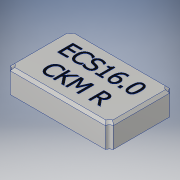
# Autodesk Inventor part: Crystal_ECX-42
Saved by Autodesk Inventor 2018 (Build 220112000, 112)
## iProperties
Created: 2016-08-15
Part Number: Crystal_ECX-42
Material: Aluminum 6061
Document SubType Name: Modeling
Designer: Bradley
Density: 2.7 g/cm^3
Appearance: Aluminum - Flat
Author: Bradley
Autodesk Inventor part; units mm, degrees
ref_plane "YZ Plane" through (0, 0, 0) normal (1, 0, 0) x (0, 1, 0)
ref_plane "XZ Plane" through (0, 0, 0) normal (0, 1, 0) x (-1, 0, 0)
ref_plane "XY Plane" through (0, 0, 0) normal (0, 0, 1) x (1, 0, 0)
sketch "Sketch1" plane through (0, 0, 0) normal (0, 1, 0) x (-1, 0, 0)
  line L0 (-2, 1.25) -> (2, 1.25)
  line L1 (2, 1.25) -> (2, -1.25)
  line L2 (2, -1.25) -> (-2, -1.25)
  line L3 (-2, -1.25) -> (-2, 1.25)
  line L4 (-2, 1.25) -> (2, -1.25) construction
  line L5 (2, 1.25) -> (-2, -1.25) construction
  arc A0 (2, -1.1) -> (1.85, -1.25) centre (2, -1.25) ccw
  arc A1 (-1.85, -1.25) -> (-2, -1.1) centre (-2, -1.25) ccw
  arc A2 (-2, 1.1) -> (-1.85, 1.25) centre (-2, 1.25) ccw
  arc A3 (1.85, 1.25) -> (2, 1.1) centre (2, 1.25) ccw
  point P0 (0, 0)
  dimension "d0" = 4
  dimension "d1" = 2.5
  dimension "d4" = 0.15
  constraints: 12 end point, 8 point on circle, 8 point on line, 4 centre point, 4 coincident, 3 equal radius, 2 midpoint, 2 parallel, 1 horizontal, 1 perpendicular
  measures "d0" distance of L1.end L2.end
  measures "d1" distance of L0.end L1.end
  measures "d4" radius of A0
extrude "Extrusion1" add sketch "Sketch1" along normal mid plane 0.9 contours L0 A3 L1 A0 L2 A1 L3 A2
chamfer "Chamfer1" distance 0.1 angle 45 8 edges at (0, 0.45, 1.25) (-1.8939, 0.45, 1.1439) (-2, 0.45, 0) (-1.8939, 0.45, -1.1439) (0, 0.45, -1.25) (1.8939, 0.45, -1.1439) (2, 0.45, 0) (1.8939, 0.45, 1.1439)
sketch "Sketch2" plane through (0, -0.45, 0) normal (0, -1, 0) x (1, 0, 0)
  line L0 (-2, 1.1) -> (-2, -1.1) projected
  arc A0 (-1.85, -1.25) -> (-2, -1.1) centre (-2, -1.25) ccw projected
  line L1 (-1.85, -1.25) -> (1.85, -1.25) projected
  arc A1 (2, -1.1) -> (1.85, -1.25) centre (2, -1.25) ccw projected
  line L2 (2, -1.1) -> (2, 1.1) projected
  arc A2 (1.85, 1.25) -> (2, 1.1) centre (2, 1.25) ccw projected
  line L3 (1.85, 1.25) -> (-1.85, 1.25) projected
  arc A3 (-2, 1.1) -> (-1.85, 1.25) centre (-2, 1.25) ccw projected
  arc A4 (-1.85, -1.25) -> (-2, -1.1) centre (-2, -1.25) ccw projected
  line L4 (-1.9612, -1.1051) -> (-1.9, -1.0439)
  line L5 (-1.9, 1.0439) -> (-1.9612, 1.1051)
  arc A5 (-2, 1.1) -> (-1.85, 1.25) centre (-2, 1.25) ccw projected
  line L6 (-1.8551, 1.2112) -> (-1.7939, 1.15)
  line L7 (-1.7939, 1.15) -> (-1, 1.15)
  line L8 (-1, -1.15) -> (-1.7939, -1.15)
  line L9 (-1.7939, -1.15) -> (-1.8551, -1.2112)
  arc A6 (1.85, 1.25) -> (2, 1.1) centre (2, 1.25) ccw projected
  line L10 (1.8551, 1.2112) -> (1.7939, 1.15)
  line L11 (1.7939, 1.15) -> (1, 1.15)
  line L12 (1, -1.15) -> (1.7939, -1.15)
  line L13 (1.7939, -1.15) -> (1.8551, -1.2112)
  arc A7 (2, -1.1) -> (1.85, -1.25) centre (2, -1.25) ccw projected
  line L14 (1.9612, -1.1051) -> (1.9, -1.0439)
  line L15 (1.9, 1.0439) -> (1.9612, 1.1051)
  line L16 (-2, 1.25) -> (-1.8939, 1.1439) construction
  line L17 (1.85, 1.25) -> (-1.85, 1.25) construction
  line L18 (-2, -1.25) -> (-1.8939, -1.1439) construction
  line L19 (-1.9, 1.0439) -> (-1.9, 0.35)
  line L20 (-1.9, 0.35) -> (-1, 0.35)
  line L21 (-1, 0.35) -> (-1, 1.15)
  line L22 (-1.9, -1.0439) -> (-1.9, -0.35)
  line L23 (-1.9, -0.35) -> (-1, -0.35)
  line L24 (-1, -0.35) -> (-1, -1.15)
  line L25 (1.9, -1.0439) -> (1.9, -0.35)
  line L26 (1.9, -0.35) -> (1, -0.35)
  line L27 (1, -0.35) -> (1, -1.15)
  line L28 (1.9, 1.0439) -> (1.9, 0.35)
  line L29 (1.9, 0.35) -> (1, 0.35)
  line L30 (1, 1.15) -> (1, 0.35)
  point P0 (0, 0)
  dimension "d9" = 0.15
  dimension "d15" = 2
  dimension "d16" = 0.7
  dimension "d17" = 0.8
  constraints: 52 end point, 15 equal length, 15 point on circle, 9 point on line, 8 parallel, 8 perpendicular, 1 collinear, 1 vertical, 1 other
  measures "d9" distance between parallel lines of L5 L6
  measures "d15" distance between parallel lines of L30 L21
  measures "d16" distance between parallel lines of L26 L29
  measures "d17" distance of L11.end L29.end
sketch "Sketch3" plane through (0, 0.45, 0) normal (0, 1, 0) x (1, 0, 0)
  line L0 (-1.7709, 1.15) -> (1.7709, 1.15) projected
  arc A0 (-1.9, 1.0209) -> (-1.7709, 1.15) centre (-2, 1.25) ccw projected
  line L1 (-1.9, -1.0209) -> (-1.9, 1.0209) projected
  arc A1 (-1.7709, -1.15) -> (-1.9, -1.0209) centre (-2, -1.25) ccw projected
  line L2 (1.7709, -1.15) -> (-1.7709, -1.15) projected
  arc A2 (1.9, -1.0209) -> (1.7709, -1.15) centre (2, -1.25) ccw projected
  line L3 (1.9, 1.0209) -> (1.9, -1.0209) projected
  arc A3 (1.7709, 1.15) -> (1.9, 1.0209) centre (2, 1.25) ccw projected
  line L4 (1.9, 1.0209) -> (1.9, -1.0209) construction
  line L5 (1.9, 0.1868) -> (-1.9, 0.1868) construction
  line L6 (-1.4485, 0.1868) -> (-1.4485, 0.7868)
  line L7 (-1.4485, 0.7868) -> (-1.0731, 0.7868)
  line L8 (-1.0731, 0.7868) -> (-1.0731, 0.7158)
  line L9 (-1.0731, 0.7158) -> (-1.3687, 0.7158)
  line L10 (-1.3687, 0.7158) -> (-1.3687, 0.5514)
  line L11 (-1.3687, 0.5514) -> (-1.093, 0.5514)
  line L12 (-1.093, 0.5514) -> (-1.093, 0.4804)
  line L13 (-1.093, 0.4804) -> (-1.3687, 0.4804)
  line L14 (-1.3687, 0.4804) -> (-1.3687, 0.2577)
  line L15 (-1.3687, 0.2577) -> (-1.0731, 0.2577)
  line L16 (-1.0731, 0.2577) -> (-1.0731, 0.1868)
  line L17 (-1.0731, 0.1868) -> (-1.4485, 0.1868)
  spline S0 degree 2 poles (-0.7512, 0.1761) (-0.8096, 0.1761) (-0.9083, 0.2154) (-0.9442, 0.2548) knots 0 0 0 1 2 2 2
  spline S1 degree 2 poles (-0.9442, 0.2548) (-0.9802, 0.2937) (-1.0196, 0.4104) (-1.0196, 0.4863) knots 0 0 0 1 2 2 2
  spline S2 degree 2 poles (-1.0196, 0.4863) (-1.0196, 0.5616) (-0.9812, 0.6735) (-0.9447, 0.7148) knots 0 0 0 1 2 2 2
  spline S3 degree 2 poles (-0.9447, 0.7148) (-0.9088, 0.7552) (-0.8105, 0.7975) (-0.7498, 0.7975) knots 0 0 0 1 2 2 2
  spline S4 degree 2 poles (-0.7498, 0.7975) (-0.7196, 0.7975) (-0.6666, 0.7887) (-0.6442, 0.7819) knots 0 0 0 1 2 2 2
  spline S5 degree 2 poles (-0.6442, 0.7819) (-0.6248, 0.7756) (-0.5844, 0.7576) (-0.5645, 0.7469) knots 0 0 0 1 2 2 2
  line L18 (-0.5645, 0.7469) -> (-0.5645, 0.6506)
  line L19 (-0.5645, 0.6506) -> (-0.5708, 0.6506)
  spline S6 degree 2 poles (-0.5708, 0.6506) (-0.5815, 0.6603) (-0.6146, 0.6876) (-0.6384, 0.7007) knots 0 0 0 1 2 2 2
  spline S7 degree 2 poles (-0.6384, 0.7007) (-0.6613, 0.7133) (-0.7152, 0.7294) (-0.7502, 0.7294) knots 0 0 0 1 2 2 2
  spline S8 degree 2 poles (-0.7502, 0.7294) (-0.7887, 0.7294) (-0.8572, 0.6978) (-0.883, 0.6676) knots 0 0 0 1 2 2 2
  spline S9 degree 2 poles (-0.883, 0.6676) (-0.9083, 0.637) (-0.9365, 0.5441) (-0.9365, 0.4863) knots 0 0 0 1 2 2 2
  spline S10 degree 2 poles (-0.9365, 0.4863) (-0.9365, 0.4245) (-0.9068, 0.3355) (-0.881, 0.3049) knots 0 0 0 1 2 2 2
  spline S11 degree 2 poles (-0.881, 0.3049) (-0.8558, 0.2752) (-0.7882, 0.2451) (-0.7502, 0.2451) knots 0 0 0 1 2 2 2
  spline S12 degree 2 poles (-0.7502, 0.2451) (-0.7157, 0.2451) (-0.6569, 0.2621) (-0.634, 0.2748) knots 0 0 0 1 2 2 2
  spline S13 degree 2 poles (-0.634, 0.2748) (-0.6122, 0.2874) (-0.5796, 0.3137) (-0.5703, 0.3229) knots 0 0 0 1 2 2 2
  line L20 (-0.5703, 0.3229) -> (-0.5645, 0.3229)
  line L21 (-0.5645, 0.3229) -> (-0.5645, 0.2276)
  spline S14 degree 2 poles (-0.5645, 0.2276) (-0.5844, 0.2184) (-0.6194, 0.2013) (-0.6442, 0.1936) knots 0 0 0 1 2 2 2
  spline S15 degree 2 poles (-0.6442, 0.1936) (-0.6705, 0.1848) (-0.7152, 0.1761) (-0.7512, 0.1761) knots 0 0 0 1 2 2 2
  spline S16 degree 2 poles (-0.3229, 0.1761) (-0.388, 0.1761) (-0.4794, 0.2033) (-0.5198, 0.2227) knots 0 0 0 1 2 2 2
  line L22 (-0.5198, 0.2227) -> (-0.5198, 0.3229)
  line L23 (-0.5198, 0.3229) -> (-0.5139, 0.3229)
  spline S17 degree 2 poles (-0.5139, 0.3229) (-0.4746, 0.2859) (-0.3749, 0.2451) (-0.3287, 0.2451) knots 0 0 0 1 2 2 2
  spline S18 degree 2 poles (-0.3287, 0.2451) (-0.2626, 0.2451) (-0.195, 0.3) (-0.195, 0.3453) knots 0 0 0 1 2 2 2
  spline S19 degree 2 poles (-0.195, 0.3453) (-0.195, 0.3812) (-0.2305, 0.426) (-0.2689, 0.4372) knots 0 0 0 1 2 2 2
  spline S20 degree 2 poles (-0.2689, 0.4372) (-0.2966, 0.4449) (-0.3428, 0.4556) (-0.3773, 0.4644) knots 0 0 0 1 2 2 2
  spline S21 degree 2 poles (-0.3773, 0.4644) (-0.4084, 0.4727) (-0.4575, 0.4975) (-0.4765, 0.5174) knots 0 0 0 1 2 2 2
  spline S22 degree 2 poles (-0.4765, 0.5174) (-0.495, 0.5373) (-0.5154, 0.5908) (-0.5154, 0.6258) knots 0 0 0 1 2 2 2
  spline S23 degree 2 poles (-0.5154, 0.6258) (-0.5154, 0.6988) (-0.4016, 0.7975) (-0.3136, 0.7975) knots 0 0 0 1 2 2 2
  spline S24 degree 2 poles (-0.3136, 0.7975) (-0.263, 0.7975) (-0.1736, 0.7775) (-0.1352, 0.7586) knots 0 0 0 1 2 2 2
  line L24 (-0.1352, 0.7586) -> (-0.1352, 0.6633)
  line L25 (-0.1352, 0.6633) -> (-0.141, 0.6633)
  spline S25 degree 2 poles (-0.141, 0.6633) (-0.1697, 0.6895) (-0.2592, 0.7284) (-0.3083, 0.7284) knots 0 0 0 1 2 2 2
  spline S26 degree 2 poles (-0.3083, 0.7284) (-0.3637, 0.7284) (-0.4323, 0.6764) (-0.4323, 0.6341) knots 0 0 0 1 2 2 2
  spline S27 degree 2 poles (-0.4323, 0.6341) (-0.4323, 0.5962) (-0.3919, 0.5509) (-0.354, 0.5407) knots 0 0 0 1 2 2 2
  spline S28 degree 2 poles (-0.354, 0.5407) (-0.3287, 0.5339) (-0.2553, 0.5164) (-0.231, 0.5091) knots 0 0 0 1 2 2 2
  spline S29 degree 2 poles (-0.231, 0.5091) (-0.1692, 0.4902) (-0.1118, 0.4138) (-0.1118, 0.3579) knots 0 0 0 1 2 2 2
  spline S30 degree 2 poles (-0.1118, 0.3579) (-0.1118, 0.3224) (-0.1405, 0.2543) (-0.1663, 0.2305) knots 0 0 0 1 2 2 2
  spline S31 degree 2 poles (-0.1663, 0.2305) (-0.195, 0.2043) (-0.2679, 0.1761) (-0.3229, 0.1761) knots 0 0 0 1 2 2 2
  line L26 (0.2922, 0.1868) -> (-0.0005, 0.1868)
  line L27 (-0.0005, 0.1868) -> (-0.0005, 0.248)
  line L28 (-0.0005, 0.248) -> (0.1084, 0.248)
  line L29 (0.1084, 0.248) -> (0.1084, 0.6501)
  line L30 (0.1084, 0.6501) -> (-0.0005, 0.6501)
  line L31 (-0.0005, 0.6501) -> (-0.0005, 0.7051)
  spline S32 degree 2 poles (-0.0005, 0.7051) (0.0613, 0.7051) (0.1196, 0.7401) (0.1235, 0.7887) knots 0 0 0 1 2 2 2
  line L32 (0.1235, 0.7887) -> (0.1857, 0.7887)
  line L33 (0.1857, 0.7887) -> (0.1857, 0.248)
  line L34 (0.1857, 0.248) -> (0.2922, 0.248)
  line L35 (0.2922, 0.248) -> (0.2922, 0.1868)
  spline S33 degree 2 poles (0.7818, 0.3812) (0.7818, 0.3351) (0.7512, 0.2568) (0.7254, 0.2305) knots 0 0 0 1 2 2 2
  spline S34 degree 2 poles (0.7254, 0.2305) (0.6987, 0.2028) (0.6316, 0.1741) (0.5912, 0.1741) knots 0 0 0 1 2 2 2
  spline S35 degree 2 poles (0.5912, 0.1741) (0.5509, 0.1741) (0.4843, 0.2013) (0.459, 0.2286) knots 0 0 0 1 2 2 2
  spline S36 degree 2 poles (0.459, 0.2286) (0.4279, 0.2611) (0.3929, 0.3705) (0.3929, 0.4503) knots 0 0 0 1 2 2 2
  spline S37 degree 2 poles (0.3929, 0.4503) (0.3929, 0.5286) (0.425, 0.6545) (0.4585, 0.7012) knots 0 0 0 1 2 2 2
  spline S38 degree 2 poles (0.4585, 0.7012) (0.4911, 0.7469) (0.5942, 0.7979) (0.6618, 0.7979) knots 0 0 0 1 2 2 2
  spline S39 degree 2 poles (0.6618, 0.7979) (0.6817, 0.7979) (0.7167, 0.794) (0.7298, 0.7897) knots 0 0 0 1 2 2 2
  line L36 (0.7298, 0.7897) -> (0.7298, 0.7124)
  line L37 (0.7298, 0.7124) -> (0.7264, 0.7124)
  spline S40 degree 2 poles (0.7264, 0.7124) (0.7152, 0.7182) (0.6744, 0.7284) (0.6511, 0.7284) knots 0 0 0 1 2 2 2
  spline S41 degree 2 poles (0.6511, 0.7284) (0.5762, 0.7284) (0.4843, 0.6273) (0.4755, 0.5281) knots 0 0 0 1 2 2 2
  spline S42 degree 2 poles (0.4755, 0.5281) (0.5042, 0.548) (0.5645, 0.5699) (0.6005, 0.5699) knots 0 0 0 1 2 2 2
  spline S43 degree 2 poles (0.6005, 0.5699) (0.6355, 0.5699) (0.688, 0.5558) (0.7167, 0.5344) knots 0 0 0 1 2 2 2
  spline S44 degree 2 poles (0.7167, 0.5344) (0.7498, 0.5096) (0.7818, 0.4328) (0.7818, 0.3812) knots 0 0 0 1 2 2 2
  spline S45 degree 2 poles (0.7002, 0.3778) (0.7002, 0.4148) (0.6807, 0.4649) (0.6593, 0.4824) knots 0 0 0 1 2 2 2
  spline S46 degree 2 poles (0.6593, 0.4824) (0.6433, 0.495) (0.6034, 0.5033) (0.5825, 0.5033) knots 0 0 0 1 2 2 2
  spline S47 degree 2 poles (0.5825, 0.5033) (0.5543, 0.5033) (0.5013, 0.4863) (0.4755, 0.4702) knots 0 0 0 1 2 2 2
  spline S48 degree 2 poles (0.4755, 0.4702) (0.475, 0.4615) (0.4741, 0.4449) (0.4741, 0.4323) knots 0 0 0 1 2 2 2
  spline S49 degree 2 poles (0.4741, 0.4323) (0.4741, 0.3701) (0.4984, 0.2937) (0.5169, 0.2738) knots 0 0 0 1 2 2 2
  spline S50 degree 2 poles (0.5169, 0.2738) (0.5339, 0.2548) (0.5708, 0.2398) (0.5917, 0.2398) knots 0 0 0 1 2 2 2
  spline S51 degree 2 poles (0.5917, 0.2398) (0.6404, 0.2398) (0.7002, 0.3088) (0.7002, 0.3778) knots 0 0 0 1 2 2 2
  line L38 (0.9817, 0.1868) -> (0.8854, 0.1868)
  line L39 (0.8854, 0.1868) -> (0.8854, 0.3015)
  line L40 (0.8854, 0.3015) -> (0.9817, 0.3015)
  line L41 (0.9817, 0.3015) -> (0.9817, 0.1868)
  spline S52 degree 2 poles (1.4762, 0.4868) (1.4762, 0.3253) (1.3823, 0.1741) (1.2846, 0.1741) knots 0 0 0 1 2 2 2
  spline S53 degree 2 poles (1.2846, 0.1741) (1.1854, 0.1741) (1.0925, 0.3282) (1.0925, 0.4863) knots 0 0 0 1 2 2 2
  spline S54 degree 2 poles (1.0925, 0.4863) (1.0925, 0.6487) (1.1864, 0.7989) (1.2846, 0.7989) knots 0 0 0 1 2 2 2
  spline S55 degree 2 poles (1.2846, 0.7989) (1.3833, 0.7989) (1.4762, 0.6433) (1.4762, 0.4868) knots 0 0 0 1 2 2 2
  spline S56 degree 2 poles (1.3731, 0.3039) (1.3848, 0.3336) (1.3945, 0.425) (1.3945, 0.4868) knots 0 0 0 1 2 2 2
  spline S57 degree 2 poles (1.3945, 0.4868) (1.3945, 0.5485) (1.3848, 0.6394) (1.3726, 0.6701) knots 0 0 0 1 2 2 2
  spline S58 degree 2 poles (1.3726, 0.6701) (1.3605, 0.7007) (1.3182, 0.7323) (1.2846, 0.7323) knots 0 0 0 1 2 2 2
  spline S59 degree 2 poles (1.2846, 0.7323) (1.2511, 0.7323) (1.2078, 0.7007) (1.1951, 0.6691) knots 0 0 0 1 2 2 2
  spline S60 degree 2 poles (1.1951, 0.6691) (1.183, 0.6385) (1.1742, 0.5451) (1.1742, 0.4863) knots 0 0 0 1 2 2 2
  spline S61 degree 2 poles (1.1742, 0.4863) (1.1742, 0.4231) (1.182, 0.3385) (1.1947, 0.3054) knots 0 0 0 1 2 2 2
  spline S62 degree 2 poles (1.1947, 0.3054) (1.2063, 0.2743) (1.2496, 0.2407) (1.2846, 0.2407) knots 0 0 0 1 2 2 2
  spline S63 degree 2 poles (1.2846, 0.2407) (1.3177, 0.2407) (1.3609, 0.2723) (1.3731, 0.3039) knots 0 0 0 1 2 2 2
  spline S64 degree 2 poles (-0.8981, -0.8128) (-0.9564, -0.8128) (-1.0551, -0.7734) (-1.0911, -0.734) knots 0 0 0 1 2 2 2
  spline S65 degree 2 poles (-1.0911, -0.734) (-1.1271, -0.6951) (-1.1665, -0.5785) (-1.1665, -0.5026) knots 0 0 0 1 2 2 2
  spline S66 degree 2 poles (-1.1665, -0.5026) (-1.1665, -0.4272) (-1.128, -0.3154) (-1.0916, -0.2741) knots 0 0 0 1 2 2 2
  spline S67 degree 2 poles (-1.0916, -0.2741) (-1.0556, -0.2337) (-0.9574, -0.1914) (-0.8966, -0.1914) knots 0 0 0 1 2 2 2
  spline S68 degree 2 poles (-0.8966, -0.1914) (-0.8665, -0.1914) (-0.8135, -0.2002) (-0.7911, -0.207) knots 0 0 0 1 2 2 2
  spline S69 degree 2 poles (-0.7911, -0.207) (-0.7716, -0.2133) (-0.7313, -0.2313) (-0.7113, -0.242) knots 0 0 0 1 2 2 2
  line L42 (-0.7113, -0.242) -> (-0.7113, -0.3383)
  line L43 (-0.7113, -0.3383) -> (-0.7177, -0.3383)
  spline S70 degree 2 poles (-0.7177, -0.3383) (-0.7284, -0.3285) (-0.7614, -0.3013) (-0.7853, -0.2882) knots 0 0 0 1 2 2 2
  spline S71 degree 2 poles (-0.7853, -0.2882) (-0.8081, -0.2755) (-0.8621, -0.2595) (-0.8971, -0.2595) knots 0 0 0 1 2 2 2
  spline S72 degree 2 poles (-0.8971, -0.2595) (-0.9355, -0.2595) (-1.0041, -0.2911) (-1.0298, -0.3212) knots 0 0 0 1 2 2 2
  spline S73 degree 2 poles (-1.0298, -0.3212) (-1.0551, -0.3519) (-1.0833, -0.4447) (-1.0833, -0.5026) knots 0 0 0 1 2 2 2
  spline S74 degree 2 poles (-1.0833, -0.5026) (-1.0833, -0.5644) (-1.0536, -0.6533) (-1.0279, -0.684) knots 0 0 0 1 2 2 2
  spline S75 degree 2 poles (-1.0279, -0.684) (-1.0026, -0.7136) (-0.935, -0.7438) (-0.8971, -0.7438) knots 0 0 0 1 2 2 2
  spline S76 degree 2 poles (-0.8971, -0.7438) (-0.8626, -0.7438) (-0.8037, -0.7267) (-0.7809, -0.7141) knots 0 0 0 1 2 2 2
  spline S77 degree 2 poles (-0.7809, -0.7141) (-0.759, -0.7015) (-0.7264, -0.6752) (-0.7172, -0.666) knots 0 0 0 1 2 2 2
  line L44 (-0.7172, -0.666) -> (-0.7113, -0.666)
  line L45 (-0.7113, -0.666) -> (-0.7113, -0.7613)
  spline S78 degree 2 poles (-0.7113, -0.7613) (-0.7313, -0.7705) (-0.7663, -0.7875) (-0.7911, -0.7953) knots 0 0 0 1 2 2 2
  spline S79 degree 2 poles (-0.7911, -0.7953) (-0.8173, -0.8041) (-0.8621, -0.8128) (-0.8981, -0.8128) knots 0 0 0 1 2 2 2
  line L46 (-0.1994, -0.8021) -> (-0.3029, -0.8021)
  line L47 (-0.3029, -0.8021) -> (-0.5222, -0.523)
  line L48 (-0.5222, -0.523) -> (-0.5572, -0.5624)
  line L49 (-0.5572, -0.5624) -> (-0.5572, -0.8021)
  line L50 (-0.5572, -0.8021) -> (-0.637, -0.8021)
  line L51 (-0.637, -0.8021) -> (-0.637, -0.2021)
  line L52 (-0.637, -0.2021) -> (-0.5572, -0.2021)
  line L53 (-0.5572, -0.2021) -> (-0.5572, -0.4778)
  line L54 (-0.5572, -0.4778) -> (-0.3112, -0.2021)
  line L55 (-0.3112, -0.2021) -> (-0.2139, -0.2021)
  line L56 (-0.2139, -0.2021) -> (-0.4624, -0.47)
  line L57 (-0.4624, -0.47) -> (-0.1994, -0.8021)
  line L58 (0.3627, -0.8021) -> (0.283, -0.8021)
  line L59 (0.283, -0.8021) -> (0.283, -0.2853)
  line L60 (0.283, -0.2853) -> (0.1264, -0.6368)
  line L61 (0.1264, -0.6368) -> (0.0778, -0.6368)
  line L62 (0.0778, -0.6368) -> (-0.0773, -0.2853)
  line L63 (-0.0773, -0.2853) -> (-0.0773, -0.8021)
  line L64 (-0.0773, -0.8021) -> (-0.1517, -0.8021)
  line L65 (-0.1517, -0.8021) -> (-0.1517, -0.2021)
  line L66 (-0.1517, -0.2021) -> (-0.0428, -0.2021)
  line L67 (-0.0428, -0.2021) -> (0.107, -0.5361)
  line L68 (0.107, -0.5361) -> (0.2519, -0.2021)
  line L69 (0.2519, -0.2021) -> (0.3627, -0.2021)
  line L70 (0.3627, -0.2021) -> (0.3627, -0.8021)
  line L71 (1.2063, -0.8021) -> (1.1028, -0.8021)
  line L72 (1.1028, -0.8021) -> (0.9131, -0.5634)
  line L73 (0.9131, -0.5634) -> (0.8217, -0.5634)
  line L74 (0.8217, -0.5634) -> (0.8217, -0.8021)
  line L75 (0.8217, -0.8021) -> (0.742, -0.8021)
  line L76 (0.742, -0.8021) -> (0.742, -0.2021)
  line L77 (0.742, -0.2021) -> (0.8966, -0.2021)
  spline S80 degree 2 poles (0.8966, -0.2021) (0.9481, -0.2021) (1.0177, -0.2133) (1.0493, -0.2337) knots 0 0 0 1 2 2 2
  spline S81 degree 2 poles (1.0493, -0.2337) (1.0809, -0.2541) (1.1173, -0.3178) (1.1173, -0.365) knots 0 0 0 1 2 2 2
  spline S82 degree 2 poles (1.1173, -0.365) (1.1173, -0.4306) (1.0502, -0.5196) (0.9929, -0.541) knots 0 0 0 1 2 2 2
  line L78 (0.9929, -0.541) -> (1.2063, -0.8021)
  spline S83 degree 2 poles (1.0342, -0.3713) (1.0342, -0.3451) (1.0157, -0.3047) (0.9963, -0.2916) knots 0 0 0 1 2 2 2
  spline S84 degree 2 poles (0.9963, -0.2916) (0.9793, -0.2804) (0.934, -0.2712) (0.901, -0.2712) knots 0 0 0 1 2 2 2
  line L79 (0.901, -0.2712) -> (0.8217, -0.2712)
  line L80 (0.8217, -0.2712) -> (0.8217, -0.4968)
  line L81 (0.8217, -0.4968) -> (0.8917, -0.4968)
  spline S85 degree 2 poles (0.8917, -0.4968) (0.9263, -0.4968) (0.9812, -0.4846) (1.0002, -0.4656) knots 0 0 0 1 2 2 2
  spline S86 degree 2 poles (1.0002, -0.4656) (1.0177, -0.4491) (1.0342, -0.4024) (1.0342, -0.3713) knots 0 0 0 1 2 2 2
  point P0 (0, 0)
  constraints: 2 end point, 2 point on line, 1 horizontal, 1 perpendicular
extrude "Extrusion3" add sketch "Sketch3" along normal blind 0.01 contours L6 L7 L8 L9 L10 L11 L12 L13 L14 L15 L16 L17 | S0 S1 S2 S3 S4 S5 L18 L19 S6 S7 S8 S9 S10 S11 S12 S13 L20 L21 S14 S15 | S16 L22 L23 S17 S18 S19 S20 S21 S22 S23 S24 L24 L25 S25 S26 S27 S28 S29 S30 S31 | L26 L27 L28 L29 L30 L31 S32 L32 L33 L34 L35 | S33 S34 S35 S36 S37 S38 S39 L36 L37 S40 S41 S42 S43 S44 | L38 L39 L40 L41 | S52 S53 S54 S55 | S64 S65 S66 S67 S68 S69 L42 L43 S70 S71 S72 S73 S74 S75 S76 S77 L44 L45 S78 S79 | L46 L47 L48 L49 L50 L51 L52 L53 L54 L55 L56 L57 | L58 L59 L60 L61 L62 L63 L64 L65 L66 L67 L68 L69 L70 | L71 L72 L73 L74 L75 L76 L77 S80 S81 S82 L78
extrude "Extrusion4" add sketch "Sketch2" along normal blind 0.01 contours A3 L6 L7 L21 L20 L19 L5 | L4 L22 L23 L24 L8 L9 A0 | A2 L15 L28 L29 L30 L11 L10 | L13 L12 L27 L26 L25 L14 A1
body "Solid1"
